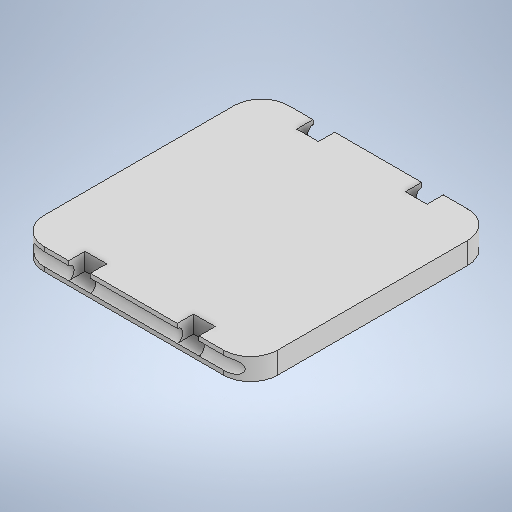
# Autodesk Inventor part: PCB_Mount
Saved by Autodesk Inventor 2025.2 (Build 292293000, 293)
## iProperties
Created: 2024-11-12
Part Number: PCB_Mount
Material: Generic
Document SubType Name: Modeling
Designer: matss
Density: 1 g/cm^3
Appearance: Default
Author: matss
Autodesk Inventor part; units mm, degrees
ref_plane "YZ Plane" through (0, 0, 0) normal (1, 0, 0) x (0, 1, 0)
ref_plane "XZ Plane" through (0, 0, 0) normal (0, 1, 0) x (-1, 0, 0)
ref_plane "XY Plane" through (0, 0, 0) normal (0, 0, 1) x (1, 0, 0)
sketch "Sketch1" plane through (0, 0, 0) normal (0, 1, 0) x (-1, 0, 0)
  line L0 (0, 14.23) -> (0, -14.23) construction
  circle A0 centre (0, 14.23) radius 1
  circle A1 centre (0, -14.23) radius 1
  line L1 (10, 22.5) -> (-33, 22.5)
  line L2 (-33, 22.5) -> (-33, -22.5)
  line L3 (-33, -22.5) -> (10, -22.5)
  line L4 (10, -22.5) -> (10, 22.5)
  point P0 (0, 0)
  point P1 (0, 0)
  point P2 (10, 0)
  dimension "d0" = 28.46
  dimension "d1" = 2
  dimension "d2" = 2
  dimension "d3" = 45
  dimension "d4" = 43
  dimension "d5" = 10
  constraints: 10 end point, 3 coincident, 2 centre point, 2 midpoint, 2 parallel, 1 horizontal, 1 horizontal alignment, 1 perpendicular
  measures "d0" distance of L0.start L0.end
  measures "d1" diameter of A0
  measures "d2" diameter of A1
  measures "d3" distance of L3.end L1.start
  measures "d4" distance between parallel lines of L2 L4
  measures "d5" distance between parallel lines of L0 L4
extrude "Extrusion1" add sketch "Sketch1" along normal blind 4 contours A0 | A1 | L4 L3 L2 L1
extrude "Extrusion2" add sketch "Sketch1" against normal blind 5 contours A0 | A1
sketch "Sketch2" plane through (0, 0, 0) normal (0, -1, 0) x (1, 0, 0)
  line L0 (19, -7.5) -> (24, -7.5)
  line L1 (24, -7.5) -> (24, -2.5)
  line L2 (24, -2.5) -> (19, -2.5)
  line L3 (19, -2.5) -> (19, -7.5)
  line L4 (33, 22.5) -> (33, -22.5) projected
  line L5 (33, -22.5) -> (-10, -22.5) projected
  point P0 (0, 0)
  dimension "d10" = 5
  dimension "d11" = 5
  dimension "d12" = 9
  dimension "d13" = 15
  constraints: 8 end point, 2 parallel, 1 horizontal, 1 perpendicular
  measures "d10" distance of L2.end L0.start
  measures "d11" distance of L0.start L0.end
  measures "d12" distance between parallel lines of L4 L1
  measures "d13" distance between parallel lines of L5 L0
extrude "Extrusion3" add sketch "Sketch2" along normal blind 2.5
sketch "Sketch3" plane through (0, 0, 0) normal (0, -1, 0) x (1, 0, 0)
  line L0 (-1, -5) -> (1, -5)
  line L1 (1, -5) -> (1, 5)
  line L2 (1, 5) -> (-1, 5)
  line L3 (-1, 5) -> (-1, -5)
  circle A0 centre (0, 14.23) radius 1 projected
  circle A1 centre (0, -14.23) radius 1 projected
  circle A2 centre (0, 14.23) radius 1 projected
  circle A3 centre (0, -14.23) radius 1 projected
  point P0 (0, 0)
  point P1 (0, -5)
  point P2 (-1, 0)
  dimension "d16" = 2
  dimension "d17" = 10
  constraints: 8 end point, 2 midpoint, 2 parallel, 1 horizontal, 1 horizontal alignment, 1 perpendicular, 1 vertical alignment
  measures "d16" distance of L1.end L2.end
  measures "d17" distance of L2.end L0.start
extrude "Extrusion4" add sketch "Sketch3" along normal blind 2.5 contours L3 L2 L1 L0
fillet "Fillet1" radius 0.5 8 edges at (-1, -1.25, -5) (1, -1.25, -5) (1, -1.25, 5) (-1, -1.25, 5) (19, -1.25, -7.5) (19, -1.25, -2.5) (24, -1.25, -7.5) (24, -1.25, -2.5)
chamfer "Chamfer2" distance 0.5 angle 45 2 edges at (1, 0, -14.23) (1, 0, 14.23)
fillet "Fillet2" radius 5 4 edges at (33, 2, -22.5) (33, 2, 22.5) (-10, 2, 22.5) (-10, 2, -22.5)
sketch "Sketch8" plane through (33, 0, 17.5) normal (1, 0, 0) x (0, 0, -1)
  line L0 (40, 0) -> (40, 4) projected
  line L1 (-5, 4) -> (-5, 0) projected
  ellipse E0 centre (40, 2) end of major axis (41, 2) minor radius 1.2
  line L2 (17.5, 0) -> (17.5, 4) construction
  line L3 (35, 4) -> (0, 4) projected
  ellipse E1 centre (-5, 2) end of major axis (-6, 2) minor radius 1.2
  dimension "d42" = 1
  dimension "d43" = 1.2
  constraints: 2 end point, 2 midpoint, 1 centre point, 1 line through centre, 1 symmetric about line, 3 other
extrude "Extrusion8" cut sketch "Sketch8" against normal blind 44.2125
sketch "Sketch9" plane through (0, 4, 0) normal (0, 1, 0) x (1, 0, 0)
  line L0 (28, 22.5) -> (-5, 22.5) projected
  line L1 (-5, -22.5) -> (28, -22.5) projected
  line L2 (11.5, 22.5) -> (11.5, -22.5) construction
  line L3 (-0.5, 22.5) -> (3.5, 22.5)
  line L4 (3.5, 22.5) -> (3.5, 19.5)
  line L5 (3.5, 19.5) -> (-0.5, 19.5)
  line L6 (-0.5, 19.5) -> (-0.5, 22.5)
  line L7 (19.5, 22.5) -> (19.5, 19.5)
  line L8 (19.5, 19.5) -> (23.5, 19.5)
  line L9 (23.5, 19.5) -> (23.5, 22.5)
  line L10 (-10, 17.5) -> (-10, -17.5) projected
  line L11 (-10, 0) -> (33, 0) construction
  line L12 (33, -17.5) -> (33, 17.5) projected
  line L13 (3.5, -22.5) -> (3.5, -19.5)
  line L14 (3.5, -19.5) -> (-0.5, -19.5)
  line L15 (-0.5, -19.5) -> (-0.5, -22.5)
  line L16 (19.5, -22.5) -> (19.5, -19.5)
  line L17 (19.5, -19.5) -> (23.5, -19.5)
  line L18 (23.5, -19.5) -> (23.5, -22.5)
  point P0 (0, 0)
  dimension "d46" = 12
  dimension "d47" = 3
  dimension "d48" = 4
  constraints: 30 end point, 12 symmetric about line, 4 midpoint, 2 parallel, 1 horizontal, 1 perpendicular, 1 point on line
  measures "d46" distance between parallel lines of L2 L6
  measures "d47" distance between parallel lines of L0 L5
  measures "d48" distance between parallel lines of L6 L4
extrude "Extrusion9" cut sketch "Sketch9" against normal blind 3.2
body "Solid1"
